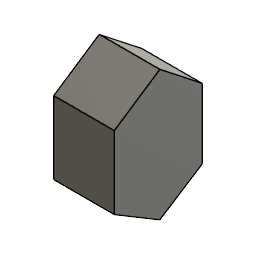
replay (Autodesk Fusion 360 design; units mm, degrees)
Autodesk Fusion 360 part; units mm, degrees
ref_plane "工作平面1" through (2, 0, 0) normal (1, 0, 0) x (0, 1, 0)
sketch "草图1" plane through (2, 0, 0) normal (1, 0, 0) x (0, 0, -1)
  line L0 (-4, 21) -> (-18, 32)
  line L1 (-18, 32) -> (-33, 22)
  line L2 (-33, 22) -> (-33, -2)
  line L3 (-33, -2) -> (-18, -11)
  line L4 (-18, -11) -> (-4, -2)
  line L5 (-4, -2) -> (-4, 21)
extrude "拉伸1" add sketch "草图1" along normal blind 20
